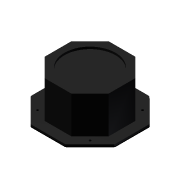
# Autodesk Inventor part: Base
Saved by Autodesk Inventor 2012 (Build 160160000, 160)
## iProperties
Created: 2013-02-21
Part Number: Base
Material: Default
Document SubType Name: Modeling
Designer: Andrew
Density: 1 g/cm^3
Author: Andrew
Autodesk Inventor part; units mm, degrees
ref_plane "YZ Plane" through (0, 0, 0) normal (1, 0, 0) x (0, 1, 0)
ref_plane "XZ Plane" through (0, 0, 0) normal (0, 1, 0) x (-1, 0, 0)
ref_plane "XY Plane" through (0, 0, 0) normal (0, 0, 1) x (1, 0, 0)
sketch "Sketch1" plane through (0, 0, 0) normal (0, 0, 1) x (1, 0, 0)
  circle A0 centre (-59.8425, -59.8526) radius 2.55
  circle A1 centre (59.8543, -59.8477) radius 2.55
  circle A2 centre (59.8494, 59.8491) radius 2.55
  circle A3 centre (-59.8474, 59.8442) radius 2.55
  arc A4 (-37.4253, 95.3527) -> (-40.9608, 93.8882) centre (-37.4253, 90.3527) ccw
  line L0 (-93.8882, 40.9608) -> (-40.9608, 93.8882)
  arc A5 (-93.8882, 40.9608) -> (-95.3527, 37.4253) centre (-90.3527, 37.4253) ccw
  line L1 (-95.3527, -37.4253) -> (-95.3527, 37.4253)
  arc A6 (-95.3527, -37.4253) -> (-93.8882, -40.9608) centre (-90.3527, -37.4253) ccw
  line L2 (-40.9608, -93.8882) -> (-93.8882, -40.9608)
  arc A7 (-40.9608, -93.8882) -> (-37.4253, -95.3527) centre (-37.4253, -90.3527) ccw
  line L3 (37.4253, -95.3527) -> (-37.4253, -95.3527)
  arc A8 (37.4253, -95.3527) -> (40.9608, -93.8882) centre (37.4253, -90.3527) ccw
  line L4 (93.8882, -40.9608) -> (40.9608, -93.8882)
  arc A9 (93.8882, -40.9608) -> (95.3527, -37.4253) centre (90.3527, -37.4253) ccw
  line L5 (95.3527, 37.4253) -> (95.3527, -37.4253)
  arc A10 (95.3527, 37.4253) -> (93.8882, 40.9608) centre (90.3527, 37.4253) ccw
  line L6 (40.9608, 93.8882) -> (93.8882, 40.9608)
  arc A11 (40.9608, 93.8882) -> (37.4253, 95.3527) centre (37.4253, 90.3527) ccw
  line L7 (-37.4253, 95.3527) -> (37.4253, 95.3527)
  circle A12 centre (55.4256, 32) radius 1.55
  circle A13 centre (55.4256, -32) radius 1.55
  circle A14 centre (0, -64) radius 1.55
  circle A15 centre (-55.4256, -32) radius 1.55
  circle A16 centre (-55.4256, 32) radius 1.55
  circle A17 centre (0, 64) radius 1.55
  arc A18 (-29.3316, 72.8127) -> (-30.7458, 72.2269) centre (-29.3316, 70.8127) ccw
  line L8 (-30.7458, 72.2269) -> (-72.2269, 30.7458)
  arc A19 (-72.2269, 30.7458) -> (-72.8127, 29.3316) centre (-70.8127, 29.3316) ccw
  line L9 (-72.8127, 29.3316) -> (-72.8127, -29.3316)
  arc A20 (-72.8127, -29.3316) -> (-72.2269, -30.7458) centre (-70.8127, -29.3316) ccw
  line L10 (-72.2269, -30.7458) -> (-30.7458, -72.2269)
  arc A21 (-30.7458, -72.2269) -> (-29.3316, -72.8127) centre (-29.3316, -70.8127) ccw
  line L11 (-29.3316, -72.8127) -> (29.3316, -72.8127)
  arc A22 (29.3316, -72.8127) -> (30.7458, -72.2269) centre (29.3316, -70.8127) ccw
  line L12 (30.7458, -72.2269) -> (72.2269, -30.7458)
  arc A23 (72.2269, -30.7458) -> (72.8127, -29.3316) centre (70.8127, -29.3316) ccw
  line L13 (72.8127, -29.3316) -> (72.8127, 29.3316)
  arc A24 (72.8127, 29.3316) -> (72.2269, 30.7458) centre (70.8127, 29.3316) ccw
  line L14 (72.2269, 30.7458) -> (30.7458, 72.2269)
  arc A25 (30.7458, 72.2269) -> (29.3316, 72.8127) centre (29.3316, 70.8127) ccw
  line L15 (29.3316, 72.8127) -> (-29.3316, 72.8127)
  circle A26 centre (0, 0) radius 58
  constraints: 16 end point, 16 point on circle, 15 centre point
extrude "Extrusion1" add sketch "Sketch1" along normal blind 4.7625 contours L7 A11 L6 A10 L5 A9 L4 A8 L3 A7 L2 A6 L1 A5 L0 A4 | A12 | A13 | A14 | A15 | A16 | A17 | L15 A25 L14 A24 L13 A23 L12 A22 L11 A21 L10 A20 L9 A19 L8 A18 | A26
extrude "Extrusion2" add sketch "Sketch1" along normal blind 89 contours A12 | A13 | A14 | A15 | A16 | A17 | L15 A25 L14 A24 L13 A23 L12 A22 L11 A21 L10 A20 L9 A19 L8 A18 | A26
sketch "Sketch2" plane through (0, 0, 89) normal (0, 0, 1) x (1, 0, 0)
  circle A0 centre (55.4256, 32) radius 1.55
  circle A1 centre (55.4256, -32) radius 1.55
  circle A2 centre (0, -64) radius 1.55
  circle A3 centre (-55.4256, -32) radius 1.55
  circle A4 centre (-55.4256, 32) radius 1.55
  circle A5 centre (0, 64) radius 1.55
  arc A6 (-29.3316, 72.8127) -> (-30.7458, 72.2269) centre (-29.3316, 70.8127) ccw
  line L0 (-30.7458, 72.2269) -> (-72.2269, 30.7458)
  arc A7 (-72.2269, 30.7458) -> (-72.8127, 29.3316) centre (-70.8127, 29.3316) ccw
  line L1 (-72.8127, 29.3316) -> (-72.8127, -29.3316)
  arc A8 (-72.8127, -29.3316) -> (-72.2269, -30.7458) centre (-70.8127, -29.3316) ccw
  line L2 (-72.2269, -30.7458) -> (-30.7458, -72.2269)
  arc A9 (-30.7458, -72.2269) -> (-29.3316, -72.8127) centre (-29.3316, -70.8127) ccw
  line L3 (-29.3316, -72.8127) -> (29.3316, -72.8127)
  arc A10 (29.3316, -72.8127) -> (30.7458, -72.2269) centre (29.3316, -70.8127) ccw
  line L4 (30.7458, -72.2269) -> (72.2269, -30.7458)
  arc A11 (72.2269, -30.7458) -> (72.8127, -29.3316) centre (70.8127, -29.3316) ccw
  line L5 (72.8127, -29.3316) -> (72.8127, 29.3316)
  arc A12 (72.8127, 29.3316) -> (72.2269, 30.7458) centre (70.8127, 29.3316) ccw
  line L6 (72.2269, 30.7458) -> (30.7458, 72.2269)
  arc A13 (30.7458, 72.2269) -> (29.3316, 72.8127) centre (29.3316, 70.8127) ccw
  line L7 (29.3316, 72.8127) -> (-29.3316, 72.8127)
  circle A14 centre (0, 0) radius 58
  point P0 (0, 0)
  constraints: 16 end point, 16 point on circle, 15 centre point
extrude "Extrusion3" cut sketch "Sketch2" against normal blind 4.7625 contours A14
body "Solid1"
